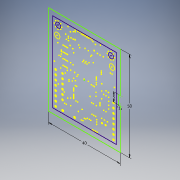
# Autodesk Inventor part: part1
Saved by Autodesk Inventor 2019 (Build 230136000, 136)
## iProperties
Created: 2020-03-18
Part Number: part1
Material: Generic
Document SubType Name: Modeling
Designer: Pulag
Density: 1 g/cm^3
Appearance: Default
Author: Pulag
Autodesk Inventor part; units mm, degrees
ref_plane "YZ Plane" through (0, 0, 0) normal (1, 0, 0) x (0, 1, 0)
ref_plane "XZ Plane" through (0, 0, 0) normal (0, 1, 0) x (-1, 0, 0)
ref_plane "XY Plane" through (0, 0, 0) normal (0, 0, 1) x (1, 0, 0)
sketch "Sketch1" plane through (0, 0, 0) normal (0, 0, 1) x (1, 0, 0)
  line L0 (-35.56, 38.35) -> (-35.56, 5)
  line L1 (0, 5) -> (0, 38.35)
  line L2 (-37.78, 47.225) -> (2.22, 47.225)
  line L3 (2.22, -2.775) -> (-37.78, -2.775)
  line L4 (-37.78, -2.775) -> (-37.78, 47.225)
  line L5 (1.22, 24.725) -> (1.22, 19.725)
  line L6 (1.22, 19.725) -> (2.22, 19.725)
  line L7 (2.22, 24.725) -> (1.22, 24.725)
  line L8 (2.22, 47.225) -> (2.22, 24.725)
  line L9 (2.22, 19.725) -> (2.22, -2.775)
  circle A0 centre (-3.05, 41.4) radius 1.4
  circle A1 centre (-32.51, 41.4) radius 1.4
  arc A2 (-6.1, 41.4) -> (-3.05, 38.35) centre (-3.05, 41.4) ccw
  line L10 (-6.1, 41.4) -> (-6.1, 44.45)
  line L11 (-3.05, 38.35) -> (0, 38.35)
  arc A3 (-32.51, 38.35) -> (-29.46, 41.4) centre (-32.51, 41.4) ccw
  line L12 (-29.46, 41.4) -> (-29.46, 44.45)
  line L13 (-32.51, 38.35) -> (-35.56, 38.35)
  line L14 (-6.1, 44.45) -> (-29.46, 44.45)
  line L15 (-35.56, 5) -> (0, 5)
  line L16 (0, 38.35) -> (0, 44.45)
  line L17 (0, 44.45) -> (-6.1, 44.45)
  line L18 (-29.46, 44.45) -> (-35.56, 44.45)
  line L19 (-35.56, 44.45) -> (-35.56, 38.35)
  line L20 (0, 5) -> (-35.56, 5)
  line L21 (-35.56, 5) -> (-35.56, -0.1476)
  line L22 (-35.56, -0.1476) -> (0, -0.1476)
  line L23 (0, -0.1476) -> (0, 5)
  point P0 (-17.78, 22.225)
  dimension "d0" = 40
  dimension "d1" = 50
  dimension "d2" = 5
  dimension "d4" = 1
  dimension "d6" = 7.775
  dimension "d8" = 3.05
  dimension "d9" = 2.8
  constraints: 48 end point, 11 perpendicular, 7 parallel, 4 centre point, 4 point on circle, 4 tangent, 3 horizontal, 2 coincident, 1 point on line, 1 vertical
  measures "d0" distance of L3.start L3.end
  measures "d1" distance of L2.end L3.start
  measures "d2" distance of L5.start L5.end
  measures "d4" distance of L5.end L6.end
  measures "d6" distance between parallel lines of L3 L15
  measures "d8" radius of A3
  measures "d9" diameter of A1
extrude "Extrusion1" add sketch "Sketch1" along normal blind 5 contours L2 L8 L7 L5 L6 L9 L3 L4
ref_plane "Work Plane1" through (0, 0, 0) normal (0, 0, 1) x (1, 0, 0)
sketch "Sketch2" plane through (0, 0, 0) normal (0, 0, 1) x (1, 0, 0)
  line L0 (-35.56, 38.35) -> (-35.56, 5)
  line L1 (0, 5) -> (0, 38.35)
  line L2 (-37.78, 47.225) -> (2.22, 47.225)
  line L3 (2.22, -2.775) -> (-37.78, -2.775)
  line L4 (-37.78, -2.775) -> (-37.78, 47.225)
  line L5 (1.22, 24.725) -> (1.22, 19.725)
  line L6 (1.22, 19.725) -> (2.22, 19.725)
  line L7 (2.22, 24.725) -> (1.22, 24.725)
  line L8 (2.22, 47.225) -> (2.22, 24.725)
  line L9 (2.22, 19.725) -> (2.22, -2.775)
  circle A0 centre (-3.05, 41.4) radius 1.4
  circle A1 centre (-32.51, 41.4) radius 1.4
  arc A2 (-6.1, 41.4) -> (-3.05, 38.35) centre (-3.05, 41.4) ccw
  line L10 (-6.1, 41.4) -> (-6.1, 44.45)
  line L11 (-3.05, 38.35) -> (0, 38.35)
  arc A3 (-32.51, 38.35) -> (-29.46, 41.4) centre (-32.51, 41.4) ccw
  line L12 (-29.46, 41.4) -> (-29.46, 44.45)
  line L13 (-32.51, 38.35) -> (-35.56, 38.35)
  line L14 (-6.1, 44.45) -> (-29.46, 44.45)
  line L15 (-35.56, 5) -> (0, 5)
  line L16 (0, 38.35) -> (0, 44.45)
  line L17 (0, 44.45) -> (-6.1, 44.45)
  line L18 (-29.46, 44.45) -> (-35.56, 44.45)
  line L19 (-35.56, 44.45) -> (-35.56, 38.35)
  line L20 (0, 5) -> (-35.56, 5)
  line L21 (-35.56, 5) -> (-35.56, -0.2)
  line L22 (-35.56, -0.2) -> (0, -0.2)
  line L23 (0, -0.2) -> (0, 5)
  line L24 (-35.56, -0.1476) -> (0, -0.1476) projected
  point P0 (0, 0)
  point P1 (-17.78, 22.225)
  dimension "d12" = 40
  dimension "d13" = 50
  dimension "d14" = 5
  dimension "d15" = 1
  dimension "d16" = 7.775
  dimension "d17" = 3.05
  dimension "d18" = 2.8
  dimension "d27" = 5.2
  constraints: 48 end point, 11 perpendicular, 7 parallel, 4 centre point, 4 point on circle, 4 tangent, 3 horizontal, 2 coincident, 1 point on line, 1 vertical
  measures "d12" distance of L3.start L3.end
  measures "d13" distance of L2.end L3.start
  measures "d14" distance of L5.start L5.end
  measures "d15" distance of L5.end L6.end
  measures "d16" distance between parallel lines of L3 L15
  measures "d17" radius of A3
  measures "d18" diameter of A1
  measures "d27" distance between parallel lines of L22 L20
extrude "Extrusion2" add sketch "Sketch2" along normal blind 2 contours L19 L18 L12 A3 L13 | L15 L23 L24 L21 | L24 L23 L22 L21 | L11 A2 L10 L17 L16
sketch "Sketch3" plane through (-37.78, -2.775, 0) normal (-1, 0, 0) x (0, 0, 1)
  line L0 (5.9421, 36.5891) -> (1.9421, 36.5891)
  line L1 (1.9421, 36.5891) -> (1.9421, 23.5891)
  line L2 (1.9421, 23.5891) -> (5.9421, 23.5891)
  line L3 (5.9421, 23.5891) -> (5.9421, 36.5891)
  point P0 (0, 2.775)
  dimension "d21" = 4
  dimension "d22" = 13
  constraints: 8 end point, 2 parallel, 1 horizontal, 1 perpendicular
  measures "d21" distance of L2.end L1.end
  measures "d22" distance of L1.end L0.end
extrude "Extrusion3" cut sketch "Sketch3" against normal up to surface (2.22 mm away)
sketch "Sketch4" plane through (0, 0, 0) normal (0, 0, -1) x (-1, 0, 0)
  line L0 (9.525, 39.121) -> (2.794, 39.121) projected
  line L1 (2.794, 39.121) -> (2.0566, 39.0072) projected
  line L2 (2.0566, 39.0072) -> (1.3738, 38.7064) projected
  arc A0 (29.46, 41.4) -> (32.51, 38.35) centre (32.51, 41.4) ccw projected
  line L3 (30.483, 39.121) -> (32.766, 39.121)
  line L4 (35.56, 38.35) -> (32.51, 38.35) projected
  arc A1 (34.63, 38.35) -> (32.766, 39.121) centre (32.5832, 36.0404) ccw
  line L5 (34.63, 38.35) -> (32.51, 38.35)
  arc A2 (30.483, 39.121) -> (32.51, 38.35) centre (32.51, 41.4) ccw
  arc A3 (3.05, 38.35) -> (6.1, 41.4) centre (3.05, 41.4) ccw projected
  arc A4 (3.05, 38.35) -> (5.1075, 39.121) centre (3.078, 41.4062) ccw
  arc A5 (2.794, 39.121) -> (0.93, 38.35) centre (2.917, 36.1849) ccw
  line L6 (5.1075, 39.121) -> (2.794, 39.121)
  line L7 (3.05, 38.35) -> (0.93, 38.35)
  point P0 (0, 0)
  constraints: 9 point on circle, 8 end point, 4 centre point, 2 concentric, 1 horizontal, 1 parallel, 1 point on line
extrude "Extrusion4" cut sketch "Sketch4" against normal blind 2 contours A4 A3 L0 | A3 L7 A5 L2 L1 L0 | L1 A5 | A5 L2 | L3 A1 L4 A0
sketch "Sketch5" plane through (0, 0, 0) normal (0, 0, -1) x (-1, 0, 0)
  line L0 (26.712, -2.7097) -> (26.628, -2.7097)
  line L1 (0, 5) -> (35.56, 5) projected
  line L2 (4.162, 5) -> (10.062, 5)
  line L3 (31.67, -2.775) -> (31.67, 5)
  line L4 (31.67, 5) -> (21.67, 5)
  line L5 (21.67, 5) -> (21.67, -2.775)
  line L6 (11.112, -2.775) -> (11.112, 5)
  line L7 (11.112, 5) -> (3.112, 5)
  line L8 (3.112, 5) -> (3.112, -2.775)
  line L9 (31.67, -2.775) -> (21.67, -2.775)
  line L10 (-2.22, -2.775) -> (37.78, -2.775) projected
  line L11 (11.112, -2.775) -> (3.112, -2.775)
  point P0 (0, 0)
  point P1 (26.67, -2.775)
  point P2 (7.112, -2.775)
  constraints: 20 end point, 2 collinear, 2 parallel, 1 horizontal, 1 point on line
extrude "Extrusion5" cut sketch "Sketch5" against normal blind 3.5 contours L1 L6 L10 L8 | L5 L1 L3 L9
sketch "Sketch6" plane through (0, 0, 0) normal (0, 0, -1) x (-1, 0, 0)
  line L0 (45.4266, 18.5636) -> (67.4266, 18.5636) projected
  line L1 (45.4266, -1.4364) -> (45.4266, 18.5636) projected
  line L2 (21.67, 3.8524) -> (21.67, -0.1476)
  line L3 (11.112, 3.8524) -> (11.112, -2.775)
  line L4 (11.112, -2.775) -> (21.67, -2.775)
  line L5 (21.67, -2.775) -> (21.67, 3.8524)
  line L6 (21.67, 3.8524) -> (11.112, 3.8524)
  line L7 (21.67, -2.775) -> (21.67, 5) projected
  point P0 (0, 0)
  dimension "d37" = 22
  dimension "d38" = 20
  constraints: 10 end point, 1 parallel, 1 perpendicular
  measures "d37" distance of L0.start L0.end
  measures "d38" distance of L1.start L0.start
extrude "Extrusion6" add sketch "Sketch6" along normal blind 2 from surface at 0
body "Solid1"
